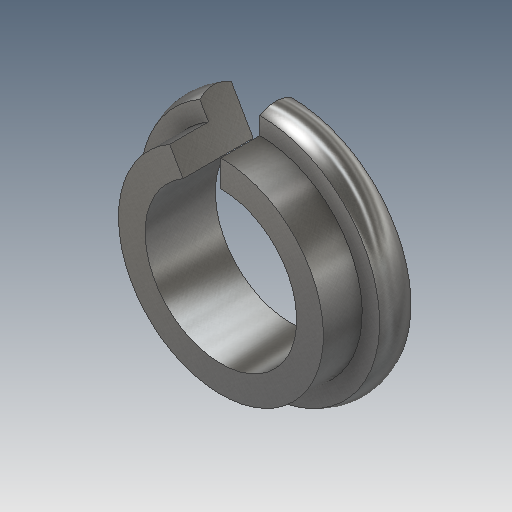
# Autodesk Inventor part: SPRING SUPPORT
Saved by Autodesk Inventor 2019 (Build 230136000, 136)
## iProperties
Created: 2023-06-18
Part Number: SPRING SUPPORT
Material: Generic
Document SubType Name: Modeling
Designer: Fransic
Density: 1 g/cm^3
Appearance: Honed
Mass: 35.6822 g
Surface Area: 115.318 cm^2
Volume: 35.6822 cm^3
Author: Fransic
Autodesk Inventor part; units mm, degrees
ref_plane "YZ Plane" through (0, 0, 0) normal (1, 0, 0) x (0, 1, 0)
ref_plane "XZ Plane" through (0, 0, 0) normal (0, 1, 0) x (-1, 0, 0)
ref_plane "XY Plane" through (0, 0, 0) normal (0, 0, 1) x (1, 0, 0)
sketch "Sketch1" plane through (0, 0, 0) normal (1, 0, 0) x (0, 1, 0)
  line L0 (0, 0) -> (0, -41.9923)
  line L1 (35.5, 0) -> (22.4345, 0)
  line L2 (22.4345, 0) -> (22.4345, -9.2803)
  line L3 (22.4345, -9.2803) -> (35.5, -9.2803)
  arc A0 (35.5, -9.2803) -> (35.5, 0) centre (27.6519, -4.6401) ccw
  constraints: 8 end point, 2 point on circle, 1 centre point, 1 horizontal, 1 parallel, 1 perpendicular, 1 vertical
revolve "Revolution1" add sketch "Sketch1" angle 330 about axis through (0, 0, 0) along (0, 0, -1)
sketch "Sketch2" plane through (0, 22.4345, 0) normal (0, 0, 1) x (1, 0, 0)
  arc A0 (-11.2172, -3.0056) -> (0, 0) centre (0, -22.4345) ccw projected
  arc A1 (-15.1658, 3.8334) -> (0, 7.8971) centre (0, -22.4345) ccw
  line L0 (-11.2172, -3.0056) -> (-15.1658, 3.8334)
  line L1 (-17.75, 8.3094) -> (-11.2172, -3.0056) projected
  line L2 (0, 7.8971) -> (0, 0)
  point P0 (0, -22.4345)
  constraints: 4 end point, 2 point on circle, 1 centre point, 1 collinear, 1 vertical
extrude "Extrusion1" add sketch "Sketch2" along normal blind 11.5
body "Solid1"
